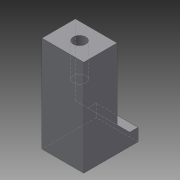
# Autodesk Inventor part: ArOZ Portable Mount
Saved by Autodesk Inventor 2015 (Build 190159000, 159)
## iProperties
Created: 2019-05-03
Part Number: ArOZ Portable Mount
Material: Generic
Document SubType Name: Modeling
Designer: Toby
Density: 1 g/cm^3
Appearance: Default
Author: Toby
Autodesk Inventor part; units mm, degrees
ref_plane "YZ Plane" through (0, 0, 0) normal (1, 0, 0) x (0, 1, 0)
ref_plane "XZ Plane" through (0, 0, 0) normal (0, 1, 0) x (-1, 0, 0)
ref_plane "XY Plane" through (0, 0, 0) normal (0, 0, 1) x (1, 0, 0)
sketch "Sketch1" plane through (0, 0, 0) normal (0, 0, 1) x (1, 0, 0)
  line L0 (-23.5606, 6.7424) -> (-13.5606, 6.7424)
  line L1 (-13.5606, 6.7424) -> (-13.5606, -1.2576)
  line L2 (-13.5606, -1.2576) -> (-23.5606, -1.2576)
  line L3 (-23.5606, -1.2576) -> (-23.5606, 6.7424)
  point P0 (0, 0)
  dimension "d0" = 10
  dimension "d1" = 8
  constraints: 8 end point, 2 parallel, 1 horizontal, 1 perpendicular
  measures "d0" distance of L0.start L0.end
  measures "d1" distance of L2.end L0.start
extrude "Extrusion1" add sketch "Sketch1" along normal blind 23
sketch "Sketch2" plane through (0, 0, 23) normal (0, 0, 1) x (1, 0, 0)
  line L0 (-23.5606, 6.7424) -> (-23.5606, -1.2576) projected
  point P0 (0, 0)
  point P1 (-18.5606, 2.7424)
  dimension "d4" = 5
  measures "d4" distance from line of L0 point (-18.561, 2.742)
hole "Hole1" at (-18.5606, 2.7424, 23) direction (0, 0, -1) diameter 3 depth 8 tip angle 118
sketch "Sketch3" plane through (-13.5606, -1.2576, 0) normal (1, 0, 0) x (0, 0, -1)
  line L0 (0, 8) -> (-3, 8)
  line L1 (-3, 8) -> (-3, 13)
  line L2 (-3, 13) -> (0, 13)
  line L3 (0, 13) -> (0, 8)
  line L4 (0, 0) -> (-23, 0) projected
  point P0 (0, 1.2576)
  dimension "d12" = 13
  dimension "d13" = 3
  constraints: 8 end point, 2 parallel, 1 horizontal, 1 perpendicular
  measures "d12" distance between parallel lines of L4 L2
  measures "d13" distance between parallel lines of L3 L1
extrude "Extrusion2" add sketch "Sketch3" against normal blind 10
chamfer "Chamfer1" distance 3 angle 45 1 edges at (-18.5606, 6.7424, 3)
body "Solid1"
